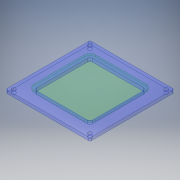
# Autodesk Inventor part: inner_tray_bottom
Saved by Autodesk Inventor 2019 (Build 230136000, 136)
## iProperties
Created: 2018-04-15
Part Number: inner_tray_bottom
Material: Generic
Document SubType Name: Modeling
Designer: cruiser
Density: 1 g/cm^3
Appearance: Clear - Green 1
Author: cruiser
Autodesk Inventor part; units mm, degrees
ref_plane "YZ Plane" through (0, 0, 0) normal (1, 0, 0) x (0, 1, 0)
ref_plane "XZ Plane" through (0, 0, 0) normal (0, 1, 0) x (-1, 0, 0)
ref_plane "XY Plane" through (0, 0, 0) normal (0, 0, 1) x (1, 0, 0)
sketch "Sketch1" plane through (0, 0, 0) normal (0, 1, 0) x (-1, 0, 0)
  line L0 (75, 75) -> (-75, 75)
  line L1 (-75, 75) -> (-75, -75)
  line L2 (-75, -75) -> (75, -75)
  line L3 (75, -75) -> (75, 75)
  line L4 (75, 75) -> (-75, -75) construction
  line L5 (-75, 75) -> (75, -75) construction
  point P0 (0, 0)
  dimension "d0" = 150
  dimension "d1" = 150
  constraints: 12 end point, 2 midpoint, 2 parallel, 1 horizontal, 1 perpendicular
  measures "d0" distance of L2.end L1.end
  measures "d1" distance of L1.end L0.end
extrude "Extrusion1" add sketch "Sketch1" along normal blind 5.88
sketch "Sketch2" plane through (0, 5.88, 0) normal (0, 1, 0) x (1, 0, 0)
  line L0 (-75.5, -90.5) -> (75.5, -90.5)
  line L1 (75.5, -90.5) -> (75.5, 90.5)
  line L2 (75.5, 90.5) -> (-75.5, 90.5)
  line L3 (-75.5, 90.5) -> (-75.5, -90.5)
  line L4 (-75.5, -90.5) -> (75.5, 90.5) construction
  line L5 (75.5, -90.5) -> (-75.5, 90.5) construction
  circle A0 centre (-68, 68) radius 3.35
  circle A1 centre (-68, -68) radius 3.35
  circle A2 centre (68, -68) radius 3.35
  circle A3 centre (68, 68) radius 3.35
  line L6 (-50, -50) -> (50, -50)
  line L7 (50, -50) -> (50, 50)
  line L8 (50, 50) -> (-50, 50)
  line L9 (-50, 50) -> (-50, -50)
  line L10 (-50, -50) -> (50, 50) construction
  line L11 (50, -50) -> (-50, 50) construction
  point P0 (0, 0)
  dimension "d4" = 151
  dimension "d5" = 181
  dimension "d6" = 6.7
  dimension "d7" = 7.5
  dimension "d8" = 22.5
  dimension "d11" = 360
  dimension "d13" = 100
  dimension "d14" = 100
  constraints: 24 end point, 4 centre point, 4 midpoint, 4 parallel, 2 horizontal, 2 perpendicular, 9 other
  measures "d4" distance of L2.end L1.end
  measures "d5" distance of L1.end L0.end
  measures "d6" diameter of A0
  measures "d7" distance from line of L3 A0.centre
  measures "d8" distance from line of L2 A0.centre
  measures "d13" distance of L8.end L7.end
  measures "d14" distance of L7.end L6.end
extrude "Extrusion2" cut sketch "Sketch2" against normal blind 5.88 contours A0 | A1 | A2 | A3 | L9 L8 L7 L6
sketch "Sketch4" plane through (0, 5.88, 0) normal (0, 1, 0) x (1, 0, 0)
  line L0 (-55, -55) -> (55, -55)
  line L1 (55, -55) -> (55, 55)
  line L2 (55, 55) -> (-55, 55)
  line L3 (-55, 55) -> (-55, -55)
  line L4 (-55, -55) -> (55, 55) construction
  line L5 (55, -55) -> (-55, 55) construction
  point P0 (0, 0)
  dimension "d21" = 110
  dimension "d22" = 110
  constraints: 12 end point, 2 midpoint, 2 parallel, 1 horizontal, 1 perpendicular
  measures "d21" distance of L2.end L1.end
  measures "d22" distance of L1.end L0.end
extrude "Extrusion4" add sketch "Sketch4" along normal blind 3.15 separate body
fillet "Fillet1" radius 10 4 edges at (-55, 7.455, 55) (55, 7.455, 55) (55, 7.455, -55) (-55, 7.455, -55)
fillet "Fillet2" radius 5 4 edges at (-50, 2.94, 50) (50, 2.94, 50) (-50, 2.94, -50) (50, 2.94, -50)
fillet "Fillet3" radius 2 4 edges at (-75, 2.94, 75) (75, 2.94, 75) (75, 2.94, -75) (-75, 2.94, -75)
equation "\"d0\" = inner_bottom_x"
equation "\"d1\" = inner_bottom_y"
equation "\"d2\" = t_inner_tray"
equation "\"d4\" = tray_x"
equation "\"d5\" = tray_y"
equation "\"d6\" = m5_brass_insert_drill"
equation "\"d7\" = 0.5 * tray_border"
equation "\"d8\" = 1.5 * tray_border"
equation "\"d13\" = bottom_clear_x - 2 * bottom_clear_border"
equation "\"d14\" = bottom_clear_y - 2 * bottom_clear_border"
equation "\"d15\" = t_inner_tray"
equation "\"d21\" = bottom_clear_x"
equation "\"d22\" = bottom_clear_y"
equation "\"d23\" = t_bottom_clear"
equation "\"d25\" = 2 * bottom_clear_border"
equation "\"d26\" = bottom_clear_border"
equation "\"d27\" = small_round"
equation "\"thick_acrylic\" = 5.88"
equation "\"thin_acrylic\" = 3.15"
equation "\"clear_acrylic\" = 3.15"
equation "\"wood_thickness\" = 6.72"
equation "\"al1_thickness\" = 1.5875"
equation "\"m3_diameter\" = 3.15"
equation "\"m4_diameter\" = 4.2"
equation "\"m5_diameter\" = 5.25"
equation "\"brass_insert_drill\" = 4"
equation "\"m5_brass_insert_drill\" = 6.7"
equation "\"m5_press_nut_drill\" = 6.35"
equation "\"m3_main_length\" = 14"
equation "\"m3_main_nut_width\" = 5.7"
equation "\"m3_main_nut_thickness\" = 2.5"
equation "\"m3_main_extra\" = 1"
equation "\"stepper_screw_space\" = 35"
equation "\"stepper_shaft_diameter\" = 5"
equation "\"stepper_body_diameter\" = 28"
equation "\"laser_body_diameter\" = 12"
equation "\"t_carrier\" = 6.72"
equation "\"t_wall\" = 5.88"
equation "\"t_window\" = 3.15"
equation "\"carrier_y\" = 181"
equation "\"carrier_z\" = 233.04"
equation "\"carrier_z2\" = 283.04"
equation "\"protection_slot\" = 30.2"
equation "\"protection_slot_offset\" = 37.75"
equation "\"protection_slot_length\" = 20.6"
equation "\"window_z\" = 185"
equation "\"window_y\" = 49.56"
equation "\"window_slot\" = 25"
equation "\"door_sensor\" = 35"
equation "\"reservoir_x\" = 151"
equation "\"reservoir_y\" = 151"
equation "\"linear_bearing_spacing\" = 207"
equation "\"linear_bearing_z\" = 304.8"
equation "\"threaded_rod_z\" = 203.2"
equation "\"motor_spacing\" = 287"
equation "\"t_tray\" = 3.15"
equation "\"tray_border\" = 15"
equation "\"tray_x\" = 151"
equation "\"tray_y\" = 181"
equation "\"bed_t\" = 1.5875"
equation "\"bed_y2\" = 45.96"
equation "\"bed_fold_x\" = 15"
equation "\"bed_gap\" = 0.3"
equation "\"t_inner_tray\" = 5.88"
equation "\"t_tape\" = 3"
equation "\"inner_tray_x\" = 145"
equation "\"inner_tray_y\" = 145"
equation "\"inner_tray_border\" = 5"
equation "\"inner_tray_radius\" = 24"
equation "\"inner_bottom_x\" = 150"
equation "\"inner_bottom_y\" = 150"
equation "\"brass_keep_out\" = 8"
equation "\"tape_keep_out\" = 2"
equation "\"tape_thickness\" = 2"
equation "\"t_crane\" = 6.72"
equation "\"crane_x\" = 244.56"
equation "\"end_stop_offset_x\" = 83"
equation "\"end_stop_spacing\" = 19"
equation "\"thumb_nut_offset_y\" = 11.72"
equation "\"thumb_nut_diameter\" = 7"
equation "\"z_min_from_center\" = 72.28"
equation "\"t_frame\" = 6.72"
equation "\"frame_top_z\" = 295"
equation "\"frame_bottom_z\" = 225"
equation "\"frame_y\" = 68.44"
equation "\"frame_border\" = 39.5"
equation "\"frame_foot_z\" = 49.5"
equation "\"frame_foot_extension\" = 6"
equation "\"frame_tilt\" = 0"
equation "\"printer_z\" = 289"
equation "\"lcd_x\" = 72"
equation "\"lcd_y\" = 25"
equation "\"subframe_y_offset\" = 27.5"
equation "\"laser_y_offset\" = 19.4"
equation "\"laser_diameter\" = 12"
equation "\"laser_z_offset\" = 55"
equation "\"laser_y\" = 33"
equation "\"laser_z\" = 33"
equation "\"laser_x\" = 62"
equation "\"t_galvo_frame\" = 6.72"
equation "\"galvo_frame_x\" = 66"
equation "\"galvo_frame_z\" = 65"
equation "\"galvo_frame_y_offset\" = 27.5"
equation "\"drawer_x\" = 181"
equation "\"drawer_y\" = 49.56"
equation "\"drawer_z\" = 206.72"
equation "\"drawer_z_from_bottom\" = 25"
equation "\"drawer_foot_mount\" = 18"
equation "\"asym_key\" = 0"
equation "\"small_round\" = 2"
equation "\"bottom_clear_x\" = 110"
equation "\"bottom_clear_y\" = 110"
equation "\"t_bottom_clear\" = 3.15"
equation "\"bottom_clear_border\" = 5"
equation "\"laser_screw_spacing_y\" = 16"
